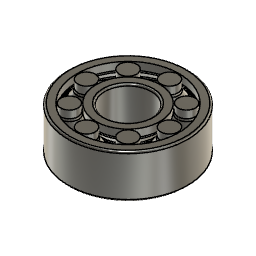
Wk4CADBearing (Autodesk Fusion 360 design; units mm, degrees)
Autodesk Fusion 360 part; units mm, degrees
sketch "Sketch1" plane through (0, 0, 0) normal (0, 0, 1) x (1, 0, 0)
  circle A0 centre (0, 0) radius 5
  dimension "d1" = 10
  constraint coincident A0.centre origin
  measures "d1" diameter of A0
extrude "Extrude1" add sketch "Sketch1" along normal blind 5 makes body 1
extrude "Extrude2" add 1 faces at (1.3101, -1.9935, 5) along direction (0, 0, 1) blind 5 draft 35 on bodies 1 bodies 1
extrude "Extrude3" add 1 faces at (2.3262, 0.6515, 10) along direction (0, 0, 1) blind 5 on bodies 1 bodies 1
extrude "Extrude4" add 1 faces at (2.3262, 0.6515, 15) along direction (0, 0, 1) blind 5 draft -35 on bodies 1 bodies 1
extrude "Extrude5" add 1 faces at (-1.0946, -1.5459, 20) along direction (0, 0, 1) blind 5 on bodies 1 bodies 1
fillet "Fillet2" radius 2 4 edges at (-7.9257, -3.0741, 15) (-4.6616, 1.8081, 20) (-7.9257, 3.0741, 10) (-4.6616, -1.8081, 5) on bodies 1
move_body "Move1" bodies 1 to x (1, 0, 0) y (0, 1, 0) z (0, 0, 1) at (-24, 0, 0)
pattern_circular "C-Pattern1" count 8 over 360 about axis through (0, 0, 1.75) along (0, 0, 1) of bodies 1 makes body 2 at (-23.5821, -14.0859, 16.8389) makes body 3 at (-6.7148, -26.6353, 16.8389) makes body 4 at (14.0859, -23.5821, 16.8389) makes body 5 at (26.6353, -6.7148, 16.8389) makes body 6 at (23.5821, 14.0859, 16.8389) makes body 7 at (6.7148, 26.6353, 16.8389) makes body 8 at (-14.0859, 23.5821, 16.8389)
sketch "Sketch2" plane through (0, 0, 0) normal (1, 0, 0) x (0, 1, 0)
  line L0 (18.5, 25) -> (18.5, 20)
  line L1 (15, 15) -> (15, 10)
  line L2 (18.5, 20) -> (15, 15)
  line L3 (18.5, 0) -> (18.5, 5)
  line L4 (18.5, 5) -> (15, 10)
  line L5 (18.5, 0) -> (13.5, 0)
  line L6 (13.5, 0) -> (13.5, 25)
  line L7 (13.5, 25) -> (18.5, 25)
  line L8 (29.5, 25) -> (29.5, 20)
  line L9 (33, 15) -> (33, 10)
  line L10 (29.5, 5) -> (29.5, 0)
  line L11 (29.5, 0) -> (34.5, 0)
  line L12 (34.5, 0) -> (34.5, 25)
  line L13 (34.5, 25) -> (29.5, 25)
  line L14 (29.5, 20) -> (33, 15)
  line L15 (33, 10) -> (29.5, 5)
  constraint vertical L0
  constraint vertical L1
  constraint vertical L3
  constraint perpendicular L3 L5
  constraint perpendicular L5 L6
  constraint perpendicular L6 L7
  constraint perpendicular L7 L8
  constraint vertical L9
  constraint vertical L10
  constraint perpendicular L10 L11
  constraint perpendicular L11 L12
  constraint perpendicular L8 L13
revolve "Revolve1" add sketch "Sketch2" angle 360 about axis through (0, 0, 1.75) along (0, 0, 1) separate body makes body 9 at (3.4351, 34.3286, 8.3333) makes body 10 at (1.3442, 13.4329, 8.3333)
fillet "Fillet1" radius 1 4 edges at (-32.1653, 12.4757, 25) (-32.1653, 12.4757, 0) (-12.5864, 4.8818, 25) (-12.5864, 4.8818, 0) on bodies 9 10
fillet "Fillet3" radius 2 4 edges at (-27.5037, 10.6677, 5) (-30.7668, 11.9333, 10) (-30.7668, 11.9333, 15) (-27.5037, 10.6677, 20) on bodies 9
fillet "Fillet4" radius 2 4 edges at (-17.2481, 6.6899, 20) (-13.9849, 5.4242, 15) (-13.9849, 5.4242, 10) (-17.2481, 6.6899, 5) on bodies 10
